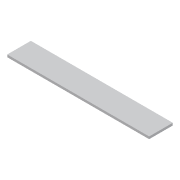
# Autodesk Inventor part: Lid_FrontPanel
Saved by Autodesk Inventor 2016 (Build 200138000, 138)
## iProperties
Created: 2014-11-24
Part Number: Lid_FrontPanel
Material: Polycarbonat, klar
Document SubType Name: Modeling
Designer: Gero Hofmann
Density: 1.2 g/cm^3
Appearance: Polycarbonat - klar
Author: Gero Hofmann
Autodesk Inventor part; units mm, degrees
ref_plane "YZ Plane" through (0, 0, 0) normal (1, 0, 0) x (0, 1, 0)
ref_plane "XZ Plane" through (0, 0, 0) normal (0, 1, 0) x (-1, 0, 0)
ref_plane "XY Plane" through (0, 0, 0) normal (0, 0, 1) x (1, 0, 0)
sketch "Skizze1" plane through (0, 0, 0) normal (0, 0, 1) x (1, 0, 0)
  line L0 (0, 0) -> (600, 0)
  line L1 (600, 0) -> (600, 100)
  line L2 (600, 100) -> (0, 100)
  line L3 (0, 100) -> (0, 0)
  dimension "d4" = 100
  dimension "d5" = 600
  constraints: 8 end point, 2 parallel, 1 horizontal, 1 perpendicular
  measures "d4" distance of L2.end L0.start
  measures "d5" distance of L0.start L0.end
extrude "Extrusion1" add sketch "Skizze1" along normal blind 10
